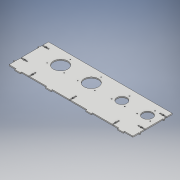
# Autodesk Inventor part: P2
Saved by Autodesk Inventor 2018 (Build 220112000, 112)
## iProperties
Created: 2018-02-28
Part Number: P2
Material: Generic
Document SubType Name: Modeling
Designer: isai
Density: 1 g/cm^3
Appearance: Default
Author: isai
Autodesk Inventor part; units mm, degrees
sketch "Sketch1" plane through (0, 0, 0) normal (0, 0, 1) x (1, 0, 0)
  line L0 (440, 140) -> (0, 140)
  line L1 (0, 140) -> (0, 0)
  line L2 (0, 0) -> (440, 0)
  line L3 (440, 0) -> (440, 140)
  circle A0 centre (402, 90) radius 18
  circle A1 centre (311, 90) radius 18
  circle A2 centre (202, 90) radius 25.5
  circle A3 centre (93, 90) radius 25.5
  point P0 (0, 0)
  constraints: 8 end point, 4 centre point
extrude "Extrusion1" add sketch "Sketch1" along normal blind 4
sketch "Sketch2" plane through (0, 0, 0) normal (0, 0, -1) x (-1, 0, 0)
  circle A0 centre (-93, 90) radius 25.5 projected
  circle A1 centre (-202, 90) radius 25.5 projected
  circle A2 centre (-311, 90) radius 18 projected
  circle A3 centre (-402, 90) radius 18 projected
  line L0 (-440, 140) -> (0, 140) projected
  line L1 (0, 140) -> (0, 0) projected
  line L2 (0, 0) -> (-440, 0) projected
  line L3 (-440, 0) -> (-440, 140) projected
  line L4 (0, 140) -> (4, 140)
  line L5 (4, 7.7) -> (0, 7.7)
  line L6 (4, 120) -> (-23, 120)
  line L7 (-23, 120) -> (-23, 116.4)
  line L8 (-23, 116.4) -> (4, 116.4)
  line L9 (4, 116.4) -> (4, 120)
  line L10 (-10, 115.2) -> (-13, 115.2)
  line L11 (-13, 115.2) -> (-13, 121.2)
  line L12 (-13, 121.2) -> (-10, 121.2)
  line L13 (-10, 121.2) -> (-10, 115.2)
  line L14 (-10, 115.2) -> (-13, 121.2) construction
  line L15 (-13, 115.2) -> (-10, 121.2) construction
  line L16 (4, 43.6) -> (-23, 43.6)
  line L17 (-23, 43.6) -> (-23, 40)
  line L18 (-23, 40) -> (4, 40)
  line L19 (4, 40) -> (4, 43.6)
  line L20 (-10, 38.8) -> (-13, 38.8)
  line L21 (-13, 38.8) -> (-13, 44.8)
  line L22 (-13, 44.8) -> (-10, 44.8)
  line L23 (-10, 44.8) -> (-10, 38.8)
  line L24 (-10, 38.8) -> (-13, 44.8) construction
  line L25 (-13, 38.8) -> (-10, 44.8) construction
  line L26 (4, 140) -> (4, 116.4)
  line L27 (4, 43.6) -> (4, 40)
  line L28 (0, 7.7) -> (0, 40)
  point P0 (-11.5, 118.2)
  point P1 (-11.5, 41.8)
  point P2 (0, 116.4)
  point P3 (0, 43.6)
  dimension "d2" = 4
  dimension "d3" = 27
  dimension "d4" = 3.6
  dimension "d5" = 3
  dimension "d6" = 6
  dimension "d7" = 10
  dimension "d8" = 140
  dimension "d9" = 20
  dimension "d15" = 27
  dimension "d17" = 3
  dimension "d18" = 6
  dimension "d22" = 40
  dimension "d23" = 3.6
  constraints: 50 end point, 11 parallel, 6 perpendicular, 5 horizontal, 4 midpoint, 4 point on line
  measures "d2" distance of L5.start L5.end
  measures "d3" distance of L8.end L7.end
  measures "d4" distance of L7.end L6.end
  measures "d5" distance of L11.end L12.end
  measures "d6" distance of L10.end L11.end
  measures "d7" distance between parallel lines of L1 L13
  measures "d8" distance between parallel lines of L2 L0
  measures "d9" distance between parallel lines of L6 L0
  measures "d15" distance of L18.end L17.end
  measures "d17" distance of L21.end L22.end
  measures "d18" distance of L20.end L21.end
  measures "d22" distance between parallel lines of L2 L18
  measures "d23" distance of L16.end L17.end
ref_plane "Work Plane2" through (220, 0, 0) normal (1, 0, 0) x (0, 0, -1)
extrude "Extrusion3" cut sketch "Sketch2" against normal blind 4 contours L6 L9 L8 L1 | L1 L8 L13 L6 | L13 L8 L11 L6 | L6 L11 L12 L13 | L16 L19 L18 L1 | L1 L18 L23 L16 | L13 L10 L11 L8 | L11 L8 L7 L6 | L23 L18 L21 L16 | L16 L21 L22 L23 | L23 L20 L21 L18 | L21 L18 L17 L16
ref_plane "Work Plane3" through (220, 140, 0) normal (-1, 0, 0) x (0, 0, 1)
mirror "Mirror2" about plane through (220, 140, 0) normal (-1, 0, 0) of "Extrusion3"
sketch "Sketch3" plane through (0, 0, 4) normal (0, 0, 1) x (1, 0, 0)
  line L0 (440, 140) -> (0, 140) projected
  line L1 (430, 43.6) -> (440, 43.6) projected
  line L2 (440, 43.6) -> (440, 116.4) projected
  line L3 (440, 116.4) -> (430, 116.4) projected
  line L4 (430, 116.4) -> (430, 115.2) projected
  line L5 (430, 115.2) -> (427, 115.2) projected
  line L6 (427, 115.2) -> (427, 116.4) projected
  line L7 (427, 116.4) -> (417, 116.4) projected
  line L8 (417, 116.4) -> (417, 120) projected
  line L9 (417, 120) -> (427, 120) projected
  line L10 (427, 120) -> (427, 121.2) projected
  line L11 (427, 121.2) -> (430, 121.2) projected
  line L12 (430, 121.2) -> (430, 120) projected
  line L13 (430, 120) -> (440, 120) projected
  line L14 (440, 120) -> (440, 140) projected
  line L15 (440, 140) -> (0, 140) projected
  line L16 (0, 140) -> (0, 120) projected
  line L17 (0, 120) -> (10, 120) projected
  line L18 (10, 120) -> (10, 121.2) projected
  line L19 (10, 121.2) -> (13, 121.2) projected
  line L20 (13, 121.2) -> (13, 120) projected
  line L21 (13, 120) -> (23, 120) projected
  line L22 (23, 120) -> (23, 116.4) projected
  line L23 (23, 116.4) -> (13, 116.4) projected
  line L24 (13, 116.4) -> (13, 115.2) projected
  line L25 (13, 115.2) -> (10, 115.2) projected
  line L26 (10, 115.2) -> (10, 116.4) projected
  line L27 (10, 116.4) -> (0, 116.4) projected
  line L28 (0, 116.4) -> (0, 43.6) projected
  line L29 (0, 43.6) -> (10, 43.6) projected
  line L30 (10, 43.6) -> (10, 44.8) projected
  line L31 (10, 44.8) -> (13, 44.8) projected
  line L32 (13, 44.8) -> (13, 43.6) projected
  line L33 (13, 43.6) -> (23, 43.6) projected
  line L34 (23, 43.6) -> (23, 40) projected
  line L35 (23, 40) -> (13, 40) projected
  line L36 (13, 40) -> (13, 38.8) projected
  line L37 (13, 38.8) -> (10, 38.8) projected
  line L38 (10, 38.8) -> (10, 40) projected
  line L39 (10, 40) -> (0, 40) projected
  line L40 (0, 40) -> (0, 0) projected
  line L41 (0, 0) -> (440, 0) projected
  line L42 (440, 0) -> (440, 40) projected
  line L43 (440, 40) -> (430, 40) projected
  line L44 (430, 40) -> (430, 38.8) projected
  line L45 (430, 38.8) -> (427, 38.8) projected
  line L46 (427, 38.8) -> (427, 40) projected
  line L47 (427, 40) -> (417, 40) projected
  line L48 (417, 40) -> (417, 43.6) projected
  line L49 (417, 43.6) -> (427, 43.6) projected
  line L50 (427, 43.6) -> (427, 44.8) projected
  line L51 (427, 44.8) -> (430, 44.8) projected
  line L52 (430, 44.8) -> (430, 43.6) projected
  circle A0 centre (93, 90) radius 25.5 projected
  circle A1 centre (202, 90) radius 25.5 projected
  circle A2 centre (311, 90) radius 18 projected
  circle A3 centre (402, 90) radius 18 projected
  line L53 (440, 110) -> (444, 110)
  line L54 (444, 110) -> (444, 106)
  line L55 (444, 106) -> (440, 106)
  line L56 (440, 106) -> (440, 110)
  line L57 (440, 24) -> (444, 24)
  line L58 (444, 24) -> (444, 20)
  line L59 (444, 20) -> (440, 20)
  line L60 (440, 20) -> (440, 24)
  point P0 (0, 0)
  dimension "d26" = 4
  dimension "d27" = 4
  dimension "d28" = 4
  dimension "d29" = 4
  dimension "d30" = 20
  dimension "d31" = 30
  constraints: 16 end point, 4 parallel, 2 horizontal, 2 perpendicular, 2 point on line
  measures "d26" distance of L54.end L55.end
  measures "d27" distance of L53.end L54.end
  measures "d28" distance of L58.end L59.end
  measures "d29" distance of L57.end L58.end
  measures "d30" distance between parallel lines of L59 L41
  measures "d31" distance between parallel lines of L53 L0
extrude "Extrusion4" add sketch "Sketch3" against normal blind 4 contours L53 L54 L55 L2 | L57 L58 L59 L42
ref_plane "Work Plane4" through (220, 43.6, 4) normal (1, 0, 0) x (0, 0, -1)
mirror "Mirror3" about plane through (220, 43.6, 4) normal (1, 0, 0) of "Extrusion4"
sketch "Sketch4" plane through (0, 0, 4) normal (0, 0, 1) x (1, 0, 0)
  line L0 (430, 43.6) -> (440, 43.6) projected
  line L1 (440, 43.6) -> (440, 106) projected
  line L2 (440, 106) -> (444, 106) projected
  line L3 (444, 106) -> (444, 110) projected
  line L4 (444, 110) -> (440, 110) projected
  line L5 (440, 110) -> (440, 116.4) projected
  line L6 (440, 116.4) -> (430, 116.4) projected
  line L7 (430, 116.4) -> (430, 115.2) projected
  line L8 (430, 115.2) -> (427, 115.2) projected
  line L9 (427, 115.2) -> (427, 116.4) projected
  line L10 (427, 116.4) -> (417, 116.4) projected
  line L11 (417, 116.4) -> (417, 120) projected
  line L12 (417, 120) -> (427, 120) projected
  line L13 (427, 120) -> (427, 121.2) projected
  line L14 (427, 121.2) -> (430, 121.2) projected
  line L15 (430, 121.2) -> (430, 120) projected
  line L16 (430, 120) -> (440, 120) projected
  line L17 (440, 120) -> (440, 140) projected
  line L18 (440, 140) -> (0, 140) projected
  line L19 (0, 140) -> (0, 120) projected
  line L20 (0, 120) -> (10, 120) projected
  line L21 (10, 120) -> (10, 121.2) projected
  line L22 (10, 121.2) -> (13, 121.2) projected
  line L23 (13, 121.2) -> (13, 120) projected
  line L24 (13, 120) -> (23, 120) projected
  line L25 (23, 120) -> (23, 116.4) projected
  line L26 (23, 116.4) -> (13, 116.4) projected
  line L27 (13, 116.4) -> (13, 115.2) projected
  line L28 (13, 115.2) -> (10, 115.2) projected
  line L29 (10, 115.2) -> (10, 116.4) projected
  line L30 (10, 116.4) -> (0, 116.4) projected
  line L31 (0, 116.4) -> (0, 110) projected
  line L32 (-4, 110) -> (0, 110) projected
  line L33 (-4, 106) -> (-4, 110) projected
  line L34 (0, 106) -> (-4, 106) projected
  line L35 (0, 106) -> (0, 43.6) projected
  line L36 (0, 43.6) -> (10, 43.6) projected
  line L37 (10, 43.6) -> (10, 44.8) projected
  line L38 (10, 44.8) -> (13, 44.8) projected
  line L39 (13, 44.8) -> (13, 43.6) projected
  line L40 (13, 43.6) -> (23, 43.6) projected
  line L41 (23, 43.6) -> (23, 40) projected
  line L42 (23, 40) -> (13, 40) projected
  line L43 (13, 40) -> (13, 38.8) projected
  line L44 (13, 38.8) -> (10, 38.8) projected
  line L45 (10, 38.8) -> (10, 40) projected
  line L46 (10, 40) -> (0, 40) projected
  line L47 (0, 40) -> (0, 24) projected
  line L48 (-4, 24) -> (0, 24) projected
  line L49 (-4, 20) -> (-4, 24) projected
  line L50 (0, 20) -> (-4, 20) projected
  line L51 (0, 20) -> (0, 0) projected
  line L52 (0, 0) -> (440, 0) projected
  line L53 (440, 0) -> (440, 20) projected
  line L54 (440, 20) -> (444, 20) projected
  line L55 (444, 20) -> (444, 24) projected
  line L56 (444, 24) -> (440, 24) projected
  line L57 (440, 24) -> (440, 40) projected
  line L58 (440, 40) -> (430, 40) projected
  line L59 (430, 40) -> (430, 38.8) projected
  line L60 (430, 38.8) -> (427, 38.8) projected
  line L61 (427, 38.8) -> (427, 40) projected
  line L62 (427, 40) -> (417, 40) projected
  line L63 (417, 40) -> (417, 43.6) projected
  line L64 (417, 43.6) -> (427, 43.6) projected
  line L65 (427, 43.6) -> (427, 44.8) projected
  line L66 (427, 44.8) -> (430, 44.8) projected
  line L67 (430, 44.8) -> (430, 43.6) projected
  circle A0 centre (93, 90) radius 25.5 projected
  circle A1 centre (202, 90) radius 25.5 projected
  circle A2 centre (311, 90) radius 18 projected
  circle A3 centre (402, 90) radius 18 projected
  line L68 (0, 43.6) -> (10, 43.6) projected
  line L69 (0, 43.6) -> (10, 43.6)
  line L70 (10, 44.8) -> (13, 44.8) projected
  line L71 (10, 43.6) -> (10, 44.8)
  line L72 (10, 44.8) -> (13, 44.8)
  line L73 (13, 43.6) -> (13, 44.8) projected
  line L74 (13, 44.8) -> (13, 43.6)
  line L75 (13, 43.6) -> (23, 43.6)
  line L76 (23, 40) -> (13, 40)
  line L77 (13, 38.8) -> (10, 38.8) projected
  line L78 (13, 38.8) -> (10, 38.8)
  line L79 (10, 40) -> (10, 38.8) projected
  line L80 (10, 38.8) -> (10, 40)
  line L81 (0, 40) -> (10, 40) projected
  line L82 (10, 40) -> (0, 40)
  line L83 (0, 40) -> (0, 43.6)
  line L84 (13, 43.6) -> (23, 43.6) projected
  line L85 (23, 43.6) -> (23, 40) projected
  line L86 (23, 43.6) -> (23, 40)
  line L87 (13, 40) -> (13, 38.8) projected
  line L88 (13, 40) -> (13, 38.8)
  line L89 (70, 0) -> (70, 10)
  line L90 (70, 10) -> (68.8, 10)
  line L91 (68.8, 10) -> (68.8, 13)
  line L92 (68.8, 13) -> (70, 13)
  line L93 (70, 13) -> (70, 23)
  line L94 (73.6, 23) -> (73.6, 13)
  line L95 (74.8, 13) -> (74.8, 10)
  line L96 (74.8, 10) -> (73.6, 10)
  line L97 (73.6, 10) -> (73.6, 0)
  line L98 (73.6, 0) -> (70, 0)
  line L99 (70, 23) -> (73.6, 23)
  line L100 (73.6, 13) -> (74.8, 13)
  line L101 (0, 0) -> (440, 0) projected
  line L102 (366.4, 13) -> (366.4, 23)
  line L103 (365.2, 13) -> (366.4, 13)
  line L104 (366.4, 23) -> (370, 23)
  line L105 (370, 23) -> (370, 13)
  line L106 (370, 13) -> (371.2, 13)
  line L107 (366.4, 10) -> (365.2, 10)
  line L108 (365.2, 10) -> (365.2, 13)
  line L109 (371.2, 13) -> (371.2, 10)
  line L110 (371.2, 10) -> (370, 10)
  line L111 (366.4, 0) -> (366.4, 10)
  line L112 (370, 10) -> (370, 0)
  line L113 (370, 0) -> (366.4, 0)
  line L114 (214.6, 13) -> (214.6, 23)
  line L115 (213.4, 13) -> (214.6, 13)
  line L116 (214.6, 23) -> (218.2, 23)
  line L117 (218.2, 23) -> (218.2, 13)
  line L118 (218.2, 13) -> (219.4, 13)
  line L119 (214.6, 10) -> (213.4, 10)
  line L120 (213.4, 10) -> (213.4, 13)
  line L121 (219.4, 13) -> (219.4, 10)
  line L122 (219.4, 10) -> (218.2, 10)
  line L123 (214.6, 0) -> (214.6, 10)
  line L124 (218.2, 10) -> (218.2, 0)
  line L125 (218.2, 0) -> (214.6, 0)
  point P0 (76.7802, 0)
  point P1 (374.5646, 0)
  point P2 (209.3918, 0)
  dimension "d34" = 70
  dimension "d35" = 3.6
  dimension "d36" = 3.6
  dimension "d37" = 6
  dimension "d38" = 1.2
  dimension "d39" = 3
  dimension "d40" = 1.2
  dimension "d41" = 3.6
  dimension "d42" = 3.6
  dimension "d43" = 6
  dimension "d44" = 1.2
  dimension "d45" = 3
  dimension "d46" = 1.2
  dimension "d47" = 3.6
  dimension "d48" = 3.6
  dimension "d49" = 6
  dimension "d50" = 1.2
  dimension "d51" = 3
  dimension "d52" = 1.2
  dimension "d53" = 70
  dimension "d54" = 440
  dimension "d55" = 221.8
  constraints: 96 end point, 24 perpendicular, 8 equal length, 1 horizontal, 1 point on line
  measures "d34" distance between parallel lines of L89 L51
  measures "d35" distance between parallel lines of L97 L89
  measures "d36" distance between parallel lines of L94 L93
  measures "d37" distance between parallel lines of L95 L91
  measures "d38" distance between parallel lines of L91 L93
  measures "d39" distance between parallel lines of L90 L92
  measures "d40" distance between parallel lines of L89 L91
  measures "d41" distance between parallel lines of L112 L111
  measures "d42" distance between parallel lines of L105 L102
  measures "d43" distance between parallel lines of L109 L108
  measures "d44" distance between parallel lines of L108 L102
  measures "d45" distance between parallel lines of L107 L103
  measures "d46" distance between parallel lines of L111 L108
  measures "d47" distance between parallel lines of L124 L123
  measures "d48" distance between parallel lines of L117 L114
  measures "d49" distance between parallel lines of L121 L120
  measures "d50" distance between parallel lines of L120 L114
  measures "d51" distance between parallel lines of L119 L115
  measures "d52" distance between parallel lines of L123 L120
  measures "d53" distance between parallel lines of L53 L112
  measures "d54" distance between parallel lines of L53 L51
  measures "d55" distance between parallel lines of L53 L124
extrude "Extrusion5" cut sketch "Sketch4" against normal blind 10 contours L52 L111 L107 L108 L103 L102 L104 L105 L106 L109 L110 L112 | L52 L123 L119 L120 L115 L114 L116 L117 L118 L121 L122 L124 | L52 L89 L90 L91 L92 L93 L99 L94 L100 L95 L96 L97
sketch "Sketch5" plane through (0, 0, 4) normal (0, 0, 1) x (1, 0, 0)
  line L0 (0, 0) -> (70, 0) projected
  line L1 (25, 0) -> (45, 0)
  line L2 (45, 0) -> (45, -5)
  line L3 (45, -5) -> (25, -5)
  line L4 (25, -5) -> (25, 0)
  line L5 (73.6, 0) -> (214.6, 0) projected
  line L6 (134.1, 0) -> (154.1, 0)
  line L7 (154.1, 0) -> (154.1, -5)
  line L8 (154.1, -5) -> (134.1, -5)
  line L9 (134.1, -5) -> (134.1, 0)
  line L10 (218.2, 0) -> (366.4, 0) projected
  line L11 (277.1516, 0) -> (297.1516, 0)
  line L12 (297.1516, 0) -> (297.1516, -5)
  line L13 (297.1516, -5) -> (277.1516, -5)
  line L14 (277.1516, -5) -> (277.1516, 0)
  line L15 (370, 0) -> (440, 0) projected
  line L16 (390.4397, 0) -> (410.4397, 0)
  line L17 (410.4397, 0) -> (410.4397, -5)
  line L18 (410.4397, -5) -> (390.4397, -5)
  line L19 (390.4397, -5) -> (390.4397, 0)
  line L20 (0, 20) -> (0, 0) projected
  line L21 (73.6, 10) -> (73.6, 0) projected
  line L22 (214.6, 0) -> (214.6, 10) projected
  line L23 (366.4, 0) -> (366.4, 10) projected
  line L24 (218.2, 10) -> (218.2, 0) projected
  dimension "d58" = 20
  dimension "d59" = 5
  dimension "d60" = 20
  dimension "d61" = 5
  dimension "d62" = 20
  dimension "d63" = 5
  dimension "d64" = 20
  dimension "d65" = 5
  dimension "d66" = 25
  dimension "d67" = 60.5
  dimension "d68" = 141
  dimension "d69" = 148.2
  constraints: 32 end point, 8 parallel, 4 horizontal, 4 perpendicular, 4 point on line
  measures "d58" distance of L2.end L3.end
  measures "d59" distance of L1.end L2.end
  measures "d60" distance of L7.end L8.end
  measures "d61" distance of L6.end L7.end
  measures "d62" distance of L12.end L13.end
  measures "d63" distance of L11.end L12.end
  measures "d64" distance of L17.end L18.end
  measures "d65" distance of L16.end L17.end
  measures "d66" distance between parallel lines of L4 L20
  measures "d67" distance between parallel lines of L9 L21
  measures "d68" distance between parallel lines of L22 L21
  measures "d69" distance between parallel lines of L23 L24
extrude "Extrusion6" add sketch "Sketch5" against normal blind 4
sketch "Boceto7" plane through (0, 0, 4) normal (0, 0, 1) x (1, 0, 0)
  line L0 (370, 10) -> (370, 0) projected
  line L1 (370, 0) -> (390.4397, 0) projected
  line L2 (390.4397, -5) -> (390.4397, 0) projected
  line L3 (410.4397, -5) -> (390.4397, -5) projected
  line L4 (410.4397, 0) -> (410.4397, -5) projected
  line L5 (410.4397, 0) -> (440, 0) projected
  line L6 (440, 0) -> (440, 20) projected
  line L7 (440, 20) -> (444, 20) projected
  line L8 (444, 20) -> (444, 24) projected
  line L9 (444, 24) -> (440, 24) projected
  line L10 (440, 24) -> (440, 40) projected
  line L11 (440, 40) -> (430, 40) projected
  line L12 (430, 40) -> (430, 38.8) projected
  line L13 (430, 38.8) -> (427, 38.8) projected
  line L14 (427, 38.8) -> (427, 40) projected
  line L15 (427, 40) -> (417, 40) projected
  line L16 (417, 40) -> (417, 43.6) projected
  line L17 (417, 43.6) -> (427, 43.6) projected
  line L18 (427, 43.6) -> (427, 44.8) projected
  line L19 (427, 44.8) -> (430, 44.8) projected
  line L20 (430, 44.8) -> (430, 43.6) projected
  line L21 (430, 43.6) -> (440, 43.6) projected
  line L22 (440, 43.6) -> (440, 106) projected
  line L23 (440, 106) -> (444, 106) projected
  line L24 (444, 106) -> (444, 110) projected
  line L25 (444, 110) -> (440, 110) projected
  line L26 (440, 110) -> (440, 116.4) projected
  line L27 (440, 116.4) -> (430, 116.4) projected
  line L28 (430, 116.4) -> (430, 115.2) projected
  line L29 (430, 115.2) -> (427, 115.2) projected
  line L30 (427, 115.2) -> (427, 116.4) projected
  line L31 (427, 116.4) -> (417, 116.4) projected
  line L32 (417, 116.4) -> (417, 120) projected
  line L33 (417, 120) -> (427, 120) projected
  line L34 (427, 120) -> (427, 121.2) projected
  line L35 (427, 121.2) -> (430, 121.2) projected
  line L36 (430, 121.2) -> (430, 120) projected
  line L37 (430, 120) -> (440, 120) projected
  line L38 (440, 120) -> (440, 140) projected
  line L39 (440, 140) -> (0, 140) projected
  line L40 (0, 140) -> (0, 120) projected
  line L41 (0, 120) -> (10, 120) projected
  line L42 (10, 120) -> (10, 121.2) projected
  line L43 (10, 121.2) -> (13, 121.2) projected
  line L44 (13, 121.2) -> (13, 120) projected
  line L45 (13, 120) -> (23, 120) projected
  line L46 (23, 120) -> (23, 116.4) projected
  line L47 (23, 116.4) -> (13, 116.4) projected
  line L48 (13, 116.4) -> (13, 115.2) projected
  line L49 (13, 115.2) -> (10, 115.2) projected
  line L50 (10, 115.2) -> (10, 116.4) projected
  line L51 (10, 116.4) -> (0, 116.4) projected
  line L52 (0, 116.4) -> (0, 110) projected
  line L53 (-4, 110) -> (0, 110) projected
  line L54 (-4, 106) -> (-4, 110) projected
  line L55 (0, 106) -> (-4, 106) projected
  line L56 (0, 106) -> (0, 43.6) projected
  line L57 (0, 43.6) -> (10, 43.6) projected
  line L58 (10, 43.6) -> (10, 44.8) projected
  line L59 (10, 44.8) -> (13, 44.8) projected
  line L60 (13, 44.8) -> (13, 43.6) projected
  line L61 (13, 43.6) -> (23, 43.6) projected
  line L62 (23, 43.6) -> (23, 40) projected
  line L63 (23, 40) -> (13, 40) projected
  line L64 (13, 40) -> (13, 38.8) projected
  line L65 (13, 38.8) -> (10, 38.8) projected
  line L66 (10, 38.8) -> (10, 40) projected
  line L67 (10, 40) -> (0, 40) projected
  line L68 (0, 40) -> (0, 24) projected
  line L69 (-4, 24) -> (0, 24) projected
  line L70 (-4, 20) -> (-4, 24) projected
  line L71 (0, 20) -> (-4, 20) projected
  line L72 (0, 20) -> (0, 0) projected
  line L73 (0, 0) -> (25, 0) projected
  line L74 (25, -5) -> (25, 0) projected
  line L75 (45, -5) -> (25, -5) projected
  line L76 (45, 0) -> (45, -5) projected
  line L77 (45, 0) -> (70, 0) projected
  line L78 (70, 0) -> (70, 10) projected
  line L79 (70, 10) -> (68.8, 10) projected
  line L80 (68.8, 10) -> (68.8, 13) projected
  line L81 (68.8, 13) -> (70, 13) projected
  line L82 (70, 13) -> (70, 23) projected
  line L83 (70, 23) -> (73.6, 23) projected
  line L84 (73.6, 23) -> (73.6, 13) projected
  line L85 (73.6, 13) -> (74.8, 13) projected
  line L86 (74.8, 13) -> (74.8, 10) projected
  line L87 (74.8, 10) -> (73.6, 10) projected
  line L88 (73.6, 10) -> (73.6, 0) projected
  line L89 (73.6, 0) -> (134.1, 0) projected
  line L90 (134.1, -5) -> (134.1, 0) projected
  line L91 (154.1, -5) -> (134.1, -5) projected
  line L92 (154.1, 0) -> (154.1, -5) projected
  line L93 (154.1, 0) -> (214.6, 0) projected
  line L94 (214.6, 0) -> (214.6, 10) projected
  line L95 (214.6, 10) -> (213.4, 10) projected
  line L96 (213.4, 10) -> (213.4, 13) projected
  line L97 (213.4, 13) -> (214.6, 13) projected
  line L98 (214.6, 13) -> (214.6, 23) projected
  line L99 (214.6, 23) -> (218.2, 23) projected
  line L100 (218.2, 23) -> (218.2, 13) projected
  line L101 (218.2, 13) -> (219.4, 13) projected
  line L102 (219.4, 13) -> (219.4, 10) projected
  line L103 (219.4, 10) -> (218.2, 10) projected
  line L104 (218.2, 10) -> (218.2, 0) projected
  line L105 (218.2, 0) -> (277.1516, 0) projected
  line L106 (277.1516, -5) -> (277.1516, 0) projected
  line L107 (297.1516, -5) -> (277.1516, -5) projected
  line L108 (297.1516, 0) -> (297.1516, -5) projected
  line L109 (297.1516, 0) -> (366.4, 0) projected
  line L110 (366.4, 0) -> (366.4, 10) projected
  line L111 (366.4, 10) -> (365.2, 10) projected
  line L112 (365.2, 10) -> (365.2, 13) projected
  line L113 (365.2, 13) -> (366.4, 13) projected
  line L114 (366.4, 13) -> (366.4, 23) projected
  line L115 (366.4, 23) -> (370, 23) projected
  line L116 (370, 23) -> (370, 13) projected
  line L117 (370, 13) -> (371.2, 13) projected
  line L118 (371.2, 13) -> (371.2, 10) projected
  line L119 (371.2, 10) -> (370, 10) projected
  circle A0 centre (93, 90) radius 25.5 projected
  circle A1 centre (202, 90) radius 25.5 projected
  circle A2 centre (311, 90) radius 18 projected
  circle A3 centre (402, 90) radius 18 projected
  circle A4 centre (93, 90) radius 25.5
  circle A5 centre (93, 90) radius 40.5
  circle A6 centre (93, 125) radius 1.5
  circle A7 centre (62.6891, 72.5) radius 1.5
  circle A8 centre (123.3109, 72.5) radius 1.5
  line L120 (0, 40) -> (0, 24) projected
  circle A9 centre (202, 90) radius 25.5
  circle A10 centre (202, 90) radius 40.5
  circle A11 centre (202, 125) radius 1.5
  circle A12 centre (171.6891, 72.5) radius 1.5
  circle A13 centre (232.3109, 72.5) radius 1.5
  circle A14 centre (311, 90) radius 32
  circle A15 centre (311, 117) radius 1.8
  circle A16 centre (287.6173, 76.5) radius 1.8
  circle A17 centre (334.3827, 76.5) radius 1.8
  circle A18 centre (311, 90) radius 27
  circle A19 centre (402, 90) radius 32
  circle A20 centre (402, 117) radius 1.8
  circle A21 centre (378.6173, 76.5) radius 1.8
  circle A22 centre (425.3827, 76.5) radius 1.8
  circle A23 centre (402, 90) radius 27
  point P0 (0, 0)
  point P1 (93, 90)
  point P2 (0, 124.9359)
  point P3 (202, 90)
  point P4 (311, 90)
  point P5 (0, 117)
  point P6 (402, 90)
  dimension "d81" = 35
  dimension "d82" = 360
  dimension "d83" = 3
  dimension "d87" = 35
  dimension "d88" = 360
  dimension "d89" = 3
  dimension "d93" = 3.6
  dimension "d94" = 27
  dimension "d95" = 360
  dimension "d102" = 3.6
  dimension "d103" = 27
  dimension "d104" = 360
  constraints: 20 centre point, 2 point on line, 28 other
  measures "d81" distance of point (93, 90) A6.centre
  measures "d83" diameter of A6
  measures "d87" distance of point (202, 90) A11.centre
  measures "d89" diameter of A11
  measures "d93" diameter of A15
  measures "d94" distance of point (311, 90) A15.centre
  measures "d102" diameter of A20
  measures "d103" distance of point (402, 90) A20.centre
extrude "Extrusión8" cut sketch "Boceto7" against normal up to surface (4 mm away) contours A6 | A7 | A8 | A11 | A12 | A13 | A15 A18 | A18 A15 | A18 A16 | A16 A18 | A18 A17 | A17 A18 | A20 A23 | A23 A20 | A23 A21 | A21 A23 | A23 A22 | A22 A23
equation "\"d83\" = d84"
equation "\"d89\" = d90"
equation "\"d80\" = d84"
equation "\"d84\" = 3"
equation "\"d86\" = d90"
equation "\"d90\" = 3"
equation "\"d105\" = 3"
equation "\"d106\" = 3"
body "Solid1"
